Autodesk Fusion 360 part; units mm, degrees
(part 2 of 10)
sketch "Sketch15" plane through (0, 0, 9) normal (0, 0, 1) x (-1, 0, 0)
  line L0 (-13.7, 38.77) -> (-13.7, 37.77)
  line L1 (-13.7, 37.77) -> (-14.7, 37.77)
  line L2 (-14.7, 37.77) -> (-14.7, 38.77)
  line L3 (-14.7, 38.77) -> (-13.7, 38.77)
  line L4 (-13.7, 36.14) -> (-13.7, 35.14)
  line L5 (-13.7, 35.14) -> (-14.7, 35.14)
  line L6 (-14.7, 35.14) -> (-14.7, 36.14)
  line L7 (-14.7, 36.14) -> (-13.7, 36.14)
  line L8 (-13.7, 33.51) -> (-13.7, 32.51)
  line L9 (-13.7, 32.51) -> (-14.7, 32.51)
  line L10 (-14.7, 32.51) -> (-14.7, 33.51)
  line L11 (-14.7, 33.51) -> (-13.7, 33.51)
  line L12 (-13.7, 30.88) -> (-13.7, 29.88)
  line L13 (-13.7, 29.88) -> (-14.7, 29.88)
  line L14 (-14.7, 29.88) -> (-14.7, 30.88)
  line L15 (-14.7, 30.88) -> (-13.7, 30.88)
  line L16 (-13.7, 28.25) -> (-13.7, 27.25)
  line L17 (-13.7, 27.25) -> (-14.7, 27.25)
  line L18 (-14.7, 27.25) -> (-14.7, 28.25)
  line L19 (-14.7, 28.25) -> (-13.7, 28.25)
  line L20 (-13.7, 25.62) -> (-13.7, 24.62)
  line L21 (-13.7, 24.62) -> (-14.7, 24.62)
  line L22 (-14.7, 24.62) -> (-14.7, 25.62)
  line L23 (-14.7, 25.62) -> (-13.7, 25.62)
  line L24 (-13.7, 22.99) -> (-13.7, 21.99)
  line L25 (-13.7, 21.99) -> (-14.7, 21.99)
  line L26 (-14.7, 21.99) -> (-14.7, 22.99)
  line L27 (-14.7, 22.99) -> (-13.7, 22.99)
  line L28 (-13.7, 20.36) -> (-13.7, 19.36)
  line L29 (-13.7, 19.36) -> (-14.7, 19.36)
  line L30 (-14.7, 19.36) -> (-14.7, 20.36)
  line L31 (-14.7, 20.36) -> (-13.7, 20.36)
  line L32 (-13.7, 17.73) -> (-13.7, 16.73)
  line L33 (-13.7, 16.73) -> (-14.7, 16.73)
  line L34 (-14.7, 16.73) -> (-14.7, 17.73)
  line L35 (-14.7, 17.73) -> (-13.7, 17.73)
  line L36 (-13.7, 15.1) -> (-13.7, 14.1)
  line L37 (-13.7, 14.1) -> (-14.7, 14.1)
  line L38 (-14.7, 14.1) -> (-14.7, 15.1)
  line L39 (-14.7, 15.1) -> (-13.7, 15.1)
  line L40 (-13.7, 12.47) -> (-13.7, 11.47)
  line L41 (-13.7, 11.47) -> (-14.7, 11.47)
  line L42 (-14.7, 11.47) -> (-14.7, 12.47)
  line L43 (-14.7, 12.47) -> (-13.7, 12.47)
  line L44 (-13.7, 9.84) -> (-13.7, 8.84)
  line L45 (-13.7, 8.84) -> (-14.7, 8.84)
  line L46 (-14.7, 8.84) -> (-14.7, 9.84)
  line L47 (-14.7, 9.84) -> (-13.7, 9.84)
  line L48 (-13.7, 7.21) -> (-13.7, 6.21)
  line L49 (-13.7, 6.21) -> (-14.7, 6.21)
  line L50 (-14.7, 6.21) -> (-14.7, 7.21)
  line L51 (-14.7, 7.21) -> (-13.7, 7.21)
  line L52 (-13.7, 4.58) -> (-13.7, 3.58)
  line L53 (-13.7, 3.58) -> (-14.7, 3.58)
  line L54 (-14.7, 3.58) -> (-14.7, 4.58)
  line L55 (-14.7, 4.58) -> (-13.7, 4.58)
  line L56 (-13.7, 1.95) -> (-13.7, 0.95)
  line L57 (-13.7, 0.95) -> (-14.7, 0.95)
  line L58 (-14.7, 0.95) -> (-14.7, 1.95)
  line L59 (-14.7, 1.95) -> (-13.7, 1.95)
  line L60 (-13.7, -0.68) -> (-13.7, -1.68)
  line L61 (-13.7, -1.68) -> (-14.7, -1.68)
  line L62 (-14.7, -1.68) -> (-14.7, -0.68)
  line L63 (-14.7, -0.68) -> (-13.7, -0.68)
  line L64 (-13.7, -3.31) -> (-13.7, -4.31)
  line L65 (-13.7, -4.31) -> (-14.7, -4.31)
  line L66 (-14.7, -4.31) -> (-14.7, -3.31)
  line L67 (-14.7, -3.31) -> (-13.7, -3.31)
  line L68 (-13.7, -5.94) -> (-13.7, -6.94)
  line L69 (-13.7, -6.94) -> (-14.7, -6.94)
  line L70 (-14.7, -6.94) -> (-14.7, -5.94)
  line L71 (-14.7, -5.94) -> (-13.7, -5.94)
  line L72 (-13.7, -8.57) -> (-13.7, -9.57)
  line L73 (-13.7, -9.57) -> (-14.7, -9.57)
  line L74 (-14.7, -9.57) -> (-14.7, -8.57)
  line L75 (-14.7, -8.57) -> (-13.7, -8.57)
  line L76 (-13.7, -11.2) -> (-13.7, -12.2)
  line L77 (-13.7, -12.2) -> (-14.7, -12.2)
  line L78 (-14.7, -12.2) -> (-14.7, -11.2)
  line L79 (-14.7, -11.2) -> (-13.7, -11.2)
  line L80 (-13.7, -13.83) -> (-13.7, -14.83)
  line L81 (-13.7, -14.83) -> (-14.7, -14.83)
  line L82 (-14.7, -14.83) -> (-14.7, -13.83)
  line L83 (-14.7, -13.83) -> (-13.7, -13.83)
  line L84 (-13.7, -16.46) -> (-13.7, -17.46)
  line L85 (-13.7, -17.46) -> (-14.7, -17.46)
  line L86 (-14.7, -17.46) -> (-14.7, -16.46)
  line L87 (-14.7, -16.46) -> (-13.7, -16.46)
  line L88 (-13.7, -19.09) -> (-13.7, -20.09)
  line L89 (-13.7, -20.09) -> (-14.7, -20.09)
  line L90 (-14.7, -20.09) -> (-14.7, -19.09)
  line L91 (-14.7, -19.09) -> (-13.7, -19.09)
  line L92 (-13.7, -21.72) -> (-13.7, -22.72)
  line L93 (-13.7, -22.72) -> (-14.7, -22.72)
  line L94 (-14.7, -22.72) -> (-14.7, -21.72)
  line L95 (-14.7, -21.72) -> (-13.7, -21.72)
  line L96 (-13.7, -24.35) -> (-13.7, -25.35)
  line L97 (-13.7, -25.35) -> (-14.7, -25.35)
  line L98 (-14.7, -25.35) -> (-14.7, -24.35)
  line L99 (-14.7, -24.35) -> (-13.7, -24.35)
  line L100 (-13.7, -26.98) -> (-13.7, -27.98)
  line L101 (-13.7, -27.98) -> (-14.7, -27.98)
  line L102 (-14.7, -27.98) -> (-14.7, -26.98)
  line L103 (-14.7, -26.98) -> (-13.7, -26.98)
  line L104 (-13.7, -29.61) -> (-13.7, -30.61)
  line L105 (-13.7, -30.61) -> (-14.7, -30.61)
  line L106 (-14.7, -30.61) -> (-14.7, -29.61)
  line L107 (-14.7, -29.61) -> (-13.7, -29.61)
  line L108 (-13.7, -32.24) -> (-13.7, -33.24)
  line L109 (-13.7, -33.24) -> (-14.7, -33.24)
  line L110 (-14.7, -33.24) -> (-14.7, -32.24)
  line L111 (-14.7, -32.24) -> (-13.7, -32.24)
  line L112 (-13.7, -34.87) -> (-13.7, -35.87)
  line L113 (-13.7, -35.87) -> (-14.7, -35.87)
  line L114 (-14.7, -35.87) -> (-14.7, -34.87)
  line L115 (-14.7, -34.87) -> (-13.7, -34.87)
  line L116 (-13.7, -37.5) -> (-13.7, -38.5)
  line L117 (-13.7, -38.5) -> (-14.7, -38.5)
  line L118 (-14.7, -38.5) -> (-14.7, -37.5)
  line L119 (-14.7, -37.5) -> (-13.7, -37.5)
  line L120 (-10.9, 38.77) -> (-10.9, 37.77)
  line L121 (-10.9, 37.77) -> (-11.9, 37.77)
  line L122 (-11.9, 37.77) -> (-11.9, 38.77)
  line L123 (-11.9, 38.77) -> (-10.9, 38.77)
  line L124 (-10.9, 36.14) -> (-10.9, 35.14)
  line L125 (-10.9, 35.14) -> (-11.9, 35.14)
  line L126 (-11.9, 35.14) -> (-11.9, 36.14)
  line L127 (-11.9, 36.14) -> (-10.9, 36.14)
  line L128 (-10.9, 33.51) -> (-10.9, 32.51)
  line L129 (-10.9, 32.51) -> (-11.9, 32.51)
  line L130 (-11.9, 32.51) -> (-11.9, 33.51)
  line L131 (-11.9, 33.51) -> (-10.9, 33.51)
  line L132 (-10.9, 30.88) -> (-10.9, 29.88)
  line L133 (-10.9, 29.88) -> (-11.9, 29.88)
  line L134 (-11.9, 29.88) -> (-11.9, 30.88)
  line L135 (-11.9, 30.88) -> (-10.9, 30.88)
  line L136 (-10.9, 28.25) -> (-10.9, 27.25)
  line L137 (-10.9, 27.25) -> (-11.9, 27.25)
  line L138 (-11.9, 27.25) -> (-11.9, 28.25)
  line L139 (-11.9, 28.25) -> (-10.9, 28.25)
  line L140 (-10.9, 25.62) -> (-10.9, 24.62)
  line L141 (-10.9, 24.62) -> (-11.9, 24.62)
  line L142 (-11.9, 24.62) -> (-11.9, 25.62)
  line L143 (-11.9, 25.62) -> (-10.9, 25.62)
  line L144 (-10.9, 22.99) -> (-10.9, 21.99)
  line L145 (-10.9, 21.99) -> (-11.9, 21.99)
  line L146 (-11.9, 21.99) -> (-11.9, 22.99)
  line L147 (-11.9, 22.99) -> (-10.9, 22.99)
  line L148 (-10.9, 20.36) -> (-10.9, 19.36)
  line L149 (-10.9, 19.36) -> (-11.9, 19.36)
  line L150 (-11.9, 19.36) -> (-11.9, 20.36)
  line L151 (-11.9, 20.36) -> (-10.9, 20.36)
  line L152 (-10.9, 17.73) -> (-10.9, 16.73)
  line L153 (-10.9, 16.73) -> (-11.9, 16.73)
  line L154 (-11.9, 16.73) -> (-11.9, 17.73)
  line L155 (-11.9, 17.73) -> (-10.9, 17.73)
  line L156 (-10.9, 15.1) -> (-10.9, 14.1)
  line L157 (-10.9, 14.1) -> (-11.9, 14.1)
  line L158 (-11.9, 14.1) -> (-11.9, 15.1)
  line L159 (-11.9, 15.1) -> (-10.9, 15.1)
  line L160 (-10.9, 12.47) -> (-10.9, 11.47)
  line L161 (-10.9, 11.47) -> (-11.9, 11.47)
  line L162 (-11.9, 11.47) -> (-11.9, 12.47)
  line L163 (-11.9, 12.47) -> (-10.9, 12.47)
  line L164 (-10.9, 9.84) -> (-10.9, 8.84)
  line L165 (-10.9, 8.84) -> (-11.9, 8.84)
  line L166 (-11.9, 8.84) -> (-11.9, 9.84)
  line L167 (-11.9, 9.84) -> (-10.9, 9.84)
  line L168 (-10.9, 7.21) -> (-10.9, 6.21)
  line L169 (-10.9, 6.21) -> (-11.9, 6.21)
  line L170 (-11.9, 6.21) -> (-11.9, 7.21)
  line L171 (-11.9, 7.21) -> (-10.9, 7.21)
  line L172 (-10.9, 4.58) -> (-10.9, 3.58)
  line L173 (-10.9, 3.58) -> (-11.9, 3.58)
  line L174 (-11.9, 3.58) -> (-11.9, 4.58)
  line L175 (-11.9, 4.58) -> (-10.9, 4.58)
  line L176 (-10.9, 1.95) -> (-10.9, 0.95)
  line L177 (-10.9, 0.95) -> (-11.9, 0.95)
  line L178 (-11.9, 0.95) -> (-11.9, 1.95)
  line L179 (-11.9, 1.95) -> (-10.9, 1.95)
  line L180 (-10.9, -0.68) -> (-10.9, -1.68)
  line L181 (-10.9, -1.68) -> (-11.9, -1.68)
  line L182 (-11.9, -1.68) -> (-11.9, -0.68)
  line L183 (-11.9, -0.68) -> (-10.9, -0.68)
  line L184 (-10.9, -3.31) -> (-10.9, -4.31)
  line L185 (-10.9, -4.31) -> (-11.9, -4.31)
  line L186 (-11.9, -4.31) -> (-11.9, -3.31)
  line L187 (-11.9, -3.31) -> (-10.9, -3.31)
  line L188 (-10.9, -5.94) -> (-10.9, -6.94)
  line L189 (-10.9, -6.94) -> (-11.9, -6.94)
  line L190 (-11.9, -6.94) -> (-11.9, -5.94)
  line L191 (-11.9, -5.94) -> (-10.9, -5.94)
  line L192 (-10.9, -8.57) -> (-10.9, -9.57)
  line L193 (-10.9, -9.57) -> (-11.9, -9.57)
  line L194 (-11.9, -9.57) -> (-11.9, -8.57)
  line L195 (-11.9, -8.57) -> (-10.9, -8.57)
  line L196 (-10.9, -11.2) -> (-10.9, -12.2)
  line L197 (-10.9, -12.2) -> (-11.9, -12.2)
  line L198 (-11.9, -12.2) -> (-11.9, -11.2)
  line L199 (-11.9, -11.2) -> (-10.9, -11.2)
  line L200 (-10.9, -13.83) -> (-10.9, -14.83)
  line L201 (-10.9, -14.83) -> (-11.9, -14.83)
  line L202 (-11.9, -14.83) -> (-11.9, -13.83)
  line L203 (-11.9, -13.83) -> (-10.9, -13.83)
  line L204 (-10.9, -16.46) -> (-10.9, -17.46)
  line L205 (-10.9, -17.46) -> (-11.9, -17.46)
  line L206 (-11.9, -17.46) -> (-11.9, -16.46)
  line L207 (-11.9, -16.46) -> (-10.9, -16.46)
  line L208 (-10.9, -19.09) -> (-10.9, -20.09)
  line L209 (-10.9, -20.09) -> (-11.9, -20.09)
  line L210 (-11.9, -20.09) -> (-11.9, -19.09)
  line L211 (-11.9, -19.09) -> (-10.9, -19.09)
  line L212 (-10.9, -21.72) -> (-10.9, -22.72)
  line L213 (-10.9, -22.72) -> (-11.9, -22.72)
  line L214 (-11.9, -22.72) -> (-11.9, -21.72)
  line L215 (-11.9, -21.72) -> (-10.9, -21.72)
  line L216 (-10.9, -24.35) -> (-10.9, -25.35)
  line L217 (-10.9, -25.35) -> (-11.9, -25.35)
  line L218 (-11.9, -25.35) -> (-11.9, -24.35)
  line L219 (-11.9, -24.35) -> (-10.9, -24.35)
  line L220 (-10.9, -26.98) -> (-10.9, -27.98)
  line L221 (-10.9, -27.98) -> (-11.9, -27.98)
  line L222 (-11.9, -27.98) -> (-11.9, -26.98)
  line L223 (-11.9, -26.98) -> (-10.9, -26.98)
  line L224 (-10.9, -29.61) -> (-10.9, -30.61)
  line L225 (-10.9, -30.61) -> (-11.9, -30.61)
  line L226 (-11.9, -30.61) -> (-11.9, -29.61)
  line L227 (-11.9, -29.61) -> (-10.9, -29.61)
  line L228 (-10.9, -32.24) -> (-10.9, -33.24)
  line L229 (-10.9, -33.24) -> (-11.9, -33.24)
  line L230 (-11.9, -33.24) -> (-11.9, -32.24)
  line L231 (-11.9, -32.24) -> (-10.9, -32.24)
  line L232 (-10.9, -34.87) -> (-10.9, -35.87)
  line L233 (-10.9, -35.87) -> (-11.9, -35.87)
  line L234 (-11.9, -35.87) -> (-11.9, -34.87)
  line L235 (-11.9, -34.87) -> (-10.9, -34.87)
  line L236 (-10.9, -37.5) -> (-10.9, -38.5)
  line L237 (-10.9, -38.5) -> (-11.9, -38.5)
  line L238 (-11.9, -38.5) -> (-11.9, -37.5)
  line L239 (-11.9, -37.5) -> (-10.9, -37.5)
  line L240 (-8.1, 38.77) -> (-8.1, 37.77)
  line L241 (-8.1, 37.77) -> (-9.1, 37.77)
  line L242 (-9.1, 37.77) -> (-9.1, 38.77)
  line L243 (-9.1, 38.77) -> (-8.1, 38.77)
  line L244 (-8.1, 36.14) -> (-8.1, 35.14)
  line L245 (-8.1, 35.14) -> (-9.1, 35.14)
  line L246 (-9.1, 35.14) -> (-9.1, 36.14)
  line L247 (-9.1, 36.14) -> (-8.1, 36.14)
  line L248 (-8.1, 33.51) -> (-8.1, 32.51)
  line L249 (-8.1, 32.51) -> (-9.1, 32.51)
  line L250 (-9.1, 32.51) -> (-9.1, 33.51)
  line L251 (-9.1, 33.51) -> (-8.1, 33.51)
  line L252 (-8.1, 30.88) -> (-8.1, 29.88)
  line L253 (-8.1, 29.88) -> (-9.1, 29.88)
  line L254 (-9.1, 29.88) -> (-9.1, 30.88)
  line L255 (-9.1, 30.88) -> (-8.1, 30.88)
  line L256 (-8.1, 28.25) -> (-8.1, 27.25)
  line L257 (-8.1, 27.25) -> (-9.1, 27.25)
  line L258 (-9.1, 27.25) -> (-9.1, 28.25)
  line L259 (-9.1, 28.25) -> (-8.1, 28.25)
  line L260 (-8.1, 25.62) -> (-8.1, 24.62)
  line L261 (-8.1, 24.62) -> (-9.1, 24.62)
  line L262 (-9.1, 24.62) -> (-9.1, 25.62)
  line L263 (-9.1, 25.62) -> (-8.1, 25.62)
  line L264 (-8.1, 22.99) -> (-8.1, 21.99)
  line L265 (-8.1, 21.99) -> (-9.1, 21.99)
  line L266 (-9.1, 21.99) -> (-9.1, 22.99)
  line L267 (-9.1, 22.99) -> (-8.1, 22.99)
  line L268 (-8.1, 20.36) -> (-8.1, 19.36)
  line L269 (-8.1, 19.36) -> (-9.1, 19.36)
  line L270 (-9.1, 19.36) -> (-9.1, 20.36)
  line L271 (-9.1, 20.36) -> (-8.1, 20.36)
  line L272 (-8.1, 17.73) -> (-8.1, 16.73)
  line L273 (-8.1, 16.73) -> (-9.1, 16.73)
  line L274 (-9.1, 16.73) -> (-9.1, 17.73)
  line L275 (-9.1, 17.73) -> (-8.1, 17.73)
  line L276 (-8.1, 15.1) -> (-8.1, 14.1)
  line L277 (-8.1, 14.1) -> (-9.1, 14.1)
  line L278 (-9.1, 14.1) -> (-9.1, 15.1)
  line L279 (-9.1, 15.1) -> (-8.1, 15.1)
  line L280 (-8.1, 12.47) -> (-8.1, 11.47)
  line L281 (-8.1, 11.47) -> (-9.1, 11.47)
  line L282 (-9.1, 11.47) -> (-9.1, 12.47)
  line L283 (-9.1, 12.47) -> (-8.1, 12.47)
  line L284 (-8.1, 9.84) -> (-8.1, 8.84)
  line L285 (-8.1, 8.84) -> (-9.1, 8.84)
  line L286 (-9.1, 8.84) -> (-9.1, 9.84)
  line L287 (-9.1, 9.84) -> (-8.1, 9.84)
  line L288 (-8.1, 7.21) -> (-8.1, 6.21)
  line L289 (-8.1, 6.21) -> (-9.1, 6.21)
  line L290 (-9.1, 6.21) -> (-9.1, 7.21)
  line L291 (-9.1, 7.21) -> (-8.1, 7.21)
  line L292 (-8.1, 4.58) -> (-8.1, 3.58)
  line L293 (-8.1, 3.58) -> (-9.1, 3.58)
  line L294 (-9.1, 3.58) -> (-9.1, 4.58)
  line L295 (-9.1, 4.58) -> (-8.1, 4.58)
  line L296 (-8.1, 1.95) -> (-8.1, 0.95)
  line L297 (-8.1, 0.95) -> (-9.1, 0.95)
  line L298 (-9.1, 0.95) -> (-9.1, 1.95)
  line L299 (-9.1, 1.95) -> (-8.1, 1.95)
  line L300 (-8.1, -0.68) -> (-8.1, -1.68)
  line L301 (-8.1, -1.68) -> (-9.1, -1.68)
  line L302 (-9.1, -1.68) -> (-9.1, -0.68)
  line L303 (-9.1, -0.68) -> (-8.1, -0.68)
  line L304 (-8.1, -3.31) -> (-8.1, -4.31)
  line L305 (-8.1, -4.31) -> (-9.1, -4.31)
  line L306 (-9.1, -4.31) -> (-9.1, -3.31)
  line L307 (-9.1, -3.31) -> (-8.1, -3.31)
  line L308 (-8.1, -5.94) -> (-8.1, -6.94)
  line L309 (-8.1, -6.94) -> (-9.1, -6.94)
  line L310 (-9.1, -6.94) -> (-9.1, -5.94)
  line L311 (-9.1, -5.94) -> (-8.1, -5.94)
  line L312 (-8.1, -8.57) -> (-8.1, -9.57)
  line L313 (-8.1, -9.57) -> (-9.1, -9.57)
  line L314 (-9.1, -9.57) -> (-9.1, -8.57)
  line L315 (-9.1, -8.57) -> (-8.1, -8.57)
  line L316 (-8.1, -11.2) -> (-8.1, -12.2)
  line L317 (-8.1, -12.2) -> (-9.1, -12.2)
  line L318 (-9.1, -12.2) -> (-9.1, -11.2)
  line L319 (-9.1, -11.2) -> (-8.1, -11.2)
  line L320 (-8.1, -13.83) -> (-8.1, -14.83)
  line L321 (-8.1, -14.83) -> (-9.1, -14.83)
  line L322 (-9.1, -14.83) -> (-9.1, -13.83)
  line L323 (-9.1, -13.83) -> (-8.1, -13.83)
  line L324 (-8.1, -16.46) -> (-8.1, -17.46)
  line L325 (-8.1, -17.46) -> (-9.1, -17.46)
  line L326 (-9.1, -17.46) -> (-9.1, -16.46)
  line L327 (-9.1, -16.46) -> (-8.1, -16.46)
  line L328 (-8.1, -19.09) -> (-8.1, -20.09)
  line L329 (-8.1, -20.09) -> (-9.1, -20.09)
  line L330 (-9.1, -20.09) -> (-9.1, -19.09)
  line L331 (-9.1, -19.09) -> (-8.1, -19.09)
  line L332 (-8.1, -21.72) -> (-8.1, -22.72)
  line L333 (-8.1, -22.72) -> (-9.1, -22.72)
  line L334 (-9.1, -22.72) -> (-9.1, -21.72)
  line L335 (-9.1, -21.72) -> (-8.1, -21.72)
  line L336 (-8.1, -24.35) -> (-8.1, -25.35)
  line L337 (-8.1, -25.35) -> (-9.1, -25.35)
  line L338 (-9.1, -25.35) -> (-9.1, -24.35)
  line L339 (-9.1, -24.35) -> (-8.1, -24.35)
  line L340 (-8.1, -26.98) -> (-8.1, -27.98)
  line L341 (-8.1, -27.98) -> (-9.1, -27.98)
  line L342 (-9.1, -27.98) -> (-9.1, -26.98)
  line L343 (-9.1, -26.98) -> (-8.1, -26.98)
  line L344 (-8.1, -29.61) -> (-8.1, -30.61)
  line L345 (-8.1, -30.61) -> (-9.1, -30.61)
  line L346 (-9.1, -30.61) -> (-9.1, -29.61)
  line L347 (-9.1, -29.61) -> (-8.1, -29.61)
  line L348 (-8.1, -32.24) -> (-8.1, -33.24)
  line L349 (-8.1, -33.24) -> (-9.1, -33.24)
  line L350 (-9.1, -33.24) -> (-9.1, -32.24)
  line L351 (-9.1, -32.24) -> (-8.1, -32.24)
  line L352 (-8.1, -34.87) -> (-8.1, -35.87)
  line L353 (-8.1, -35.87) -> (-9.1, -35.87)
  line L354 (-9.1, -35.87) -> (-9.1, -34.87)
  line L355 (-9.1, -34.87) -> (-8.1, -34.87)
  line L356 (-8.1, -37.5) -> (-8.1, -38.5)
  line L357 (-8.1, -38.5) -> (-9.1, -38.5)
  line L358 (-9.1, -38.5) -> (-9.1, -37.5)
  line L359 (-9.1, -37.5) -> (-8.1, -37.5)
  line L360 (-5.3, 38.77) -> (-5.3, 37.77)
  line L361 (-5.3, 37.77) -> (-6.3, 37.77)
  line L362 (-6.3, 37.77) -> (-6.3, 38.77)
  line L363 (-6.3, 38.77) -> (-5.3, 38.77)
  line L364 (-5.3, 36.14) -> (-5.3, 35.14)
  line L365 (-5.3, 35.14) -> (-6.3, 35.14)
  line L366 (-6.3, 35.14) -> (-6.3, 36.14)
  line L367 (-6.3, 36.14) -> (-5.3, 36.14)
  line L368 (-5.3, 33.51) -> (-5.3, 32.51)
  line L369 (-5.3, 32.51) -> (-6.3, 32.51)
  line L370 (-6.3, 32.51) -> (-6.3, 33.51)
  line L371 (-6.3, 33.51) -> (-5.3, 33.51)
  line L372 (-5.3, 30.88) -> (-5.3, 29.88)
  line L373 (-5.3, 29.88) -> (-6.3, 29.88)
  line L374 (-6.3, 29.88) -> (-6.3, 30.88)
  line L375 (-6.3, 30.88) -> (-5.3, 30.88)
  line L376 (-5.3, 28.25) -> (-5.3, 27.25)
  line L377 (-5.3, 27.25) -> (-6.3, 27.25)
  line L378 (-6.3, 27.25) -> (-6.3, 28.25)
  line L379 (-6.3, 28.25) -> (-5.3, 28.25)
  line L380 (-5.3, 25.62) -> (-5.3, 24.62)
  line L381 (-5.3, 24.62) -> (-6.3, 24.62)
  line L382 (-6.3, 24.62) -> (-6.3, 25.62)
  line L383 (-6.3, 25.62) -> (-5.3, 25.62)
  line L384 (-5.3, 22.99) -> (-5.3, 21.99)
  line L385 (-5.3, 21.99) -> (-6.3, 21.99)
  line L386 (-6.3, 21.99) -> (-6.3, 22.99)
  line L387 (-6.3, 22.99) -> (-5.3, 22.99)
  line L388 (-5.3, 20.36) -> (-5.3, 19.36)
  line L389 (-5.3, 19.36) -> (-6.3, 19.36)
  line L390 (-6.3, 19.36) -> (-6.3, 20.36)
  line L391 (-6.3, 20.36) -> (-5.3, 20.36)
  line L392 (-5.3, 17.73) -> (-5.3, 16.73)
  line L393 (-5.3, 16.73) -> (-6.3, 16.73)
  line L394 (-6.3, 16.73) -> (-6.3, 17.73)
  line L395 (-6.3, 17.73) -> (-5.3, 17.73)
  line L396 (-5.3, 15.1) -> (-5.3, 14.1)
  line L397 (-5.3, 14.1) -> (-6.3, 14.1)
  line L398 (-6.3, 14.1) -> (-6.3, 15.1)
  line L399 (-6.3, 15.1) -> (-5.3, 15.1)
  line L400 (-5.3, 12.47) -> (-5.3, 11.47)
  line L401 (-5.3, 11.47) -> (-6.3, 11.47)
  line L402 (-6.3, 11.47) -> (-6.3, 12.47)
  line L403 (-6.3, 12.47) -> (-5.3, 12.47)
  line L404 (-5.3, 9.84) -> (-5.3, 8.84)
  line L405 (-5.3, 8.84) -> (-6.3, 8.84)
  line L406 (-6.3, 8.84) -> (-6.3, 9.84)
  line L407 (-6.3, 9.84) -> (-5.3, 9.84)
  line L408 (-5.3, 7.21) -> (-5.3, 6.21)
  line L409 (-5.3, 6.21) -> (-6.3, 6.21)
  line L410 (-6.3, 6.21) -> (-6.3, 7.21)
  line L411 (-6.3, 7.21) -> (-5.3, 7.21)
  line L412 (-5.3, 4.58) -> (-5.3, 3.58)
  line L413 (-5.3, 3.58) -> (-6.3, 3.58)
  line L414 (-6.3, 3.58) -> (-6.3, 4.58)
  line L415 (-6.3, 4.58) -> (-5.3, 4.58)
  line L416 (-5.3, 1.95) -> (-5.3, 0.95)
  line L417 (-5.3, 0.95) -> (-6.3, 0.95)
  line L418 (-6.3, 0.95) -> (-6.3, 1.95)
  line L419 (-6.3, 1.95) -> (-5.3, 1.95)
  line L420 (-5.3, -0.68) -> (-5.3, -1.68)
  line L421 (-5.3, -1.68) -> (-6.3, -1.68)
  line L422 (-6.3, -1.68) -> (-6.3, -0.68)
  line L423 (-6.3, -0.68) -> (-5.3, -0.68)
  line L424 (-5.3, -3.31) -> (-5.3, -4.31)
  line L425 (-5.3, -4.31) -> (-6.3, -4.31)
  line L426 (-6.3, -4.31) -> (-6.3, -3.31)
  line L427 (-6.3, -3.31) -> (-5.3, -3.31)
  line L428 (-5.3, -5.94) -> (-5.3, -6.94)
  line L429 (-5.3, -6.94) -> (-6.3, -6.94)
  line L430 (-6.3, -6.94) -> (-6.3, -5.94)
  line L431 (-6.3, -5.94) -> (-5.3, -5.94)
  line L432 (-5.3, -8.57) -> (-5.3, -9.57)
  line L433 (-5.3, -9.57) -> (-6.3, -9.57)
  line L434 (-6.3, -9.57) -> (-6.3, -8.57)
  line L435 (-6.3, -8.57) -> (-5.3, -8.57)
  line L436 (-5.3, -11.2) -> (-5.3, -12.2)
  line L437 (-5.3, -12.2) -> (-6.3, -12.2)
  line L438 (-6.3, -12.2) -> (-6.3, -11.2)
  line L439 (-6.3, -11.2) -> (-5.3, -11.2)
  line L440 (-5.3, -13.83) -> (-5.3, -14.83)
  line L441 (-5.3, -14.83) -> (-6.3, -14.83)
  line L442 (-6.3, -14.83) -> (-6.3, -13.83)
  line L443 (-6.3, -13.83) -> (-5.3, -13.83)
  line L444 (-5.3, -16.46) -> (-5.3, -17.46)
  line L445 (-5.3, -17.46) -> (-6.3, -17.46)
  line L446 (-6.3, -17.46) -> (-6.3, -16.46)
  line L447 (-6.3, -16.46) -> (-5.3, -16.46)
  line L448 (-5.3, -19.09) -> (-5.3, -20.09)
  line L449 (-5.3, -20.09) -> (-6.3, -20.09)
  line L450 (-6.3, -20.09) -> (-6.3, -19.09)
  line L451 (-6.3, -19.09) -> (-5.3, -19.09)
  line L452 (-5.3, -21.72) -> (-5.3, -22.72)
  line L453 (-5.3, -22.72) -> (-6.3, -22.72)
  line L454 (-6.3, -22.72) -> (-6.3, -21.72)
  line L455 (-6.3, -21.72) -> (-5.3, -21.72)
  line L456 (-5.3, -24.35) -> (-5.3, -25.35)
  line L457 (-5.3, -25.35) -> (-6.3, -25.35)
  line L458 (-6.3, -25.35) -> (-6.3, -24.35)
  line L459 (-6.3, -24.35) -> (-5.3, -24.35)
  line L460 (-5.3, -26.98) -> (-5.3, -27.98)
  line L461 (-5.3, -27.98) -> (-6.3, -27.98)
  line L462 (-6.3, -27.98) -> (-6.3, -26.98)
  line L463 (-6.3, -26.98) -> (-5.3, -26.98)
  line L464 (-5.3, -29.61) -> (-5.3, -30.61)
  line L465 (-5.3, -30.61) -> (-6.3, -30.61)
  line L466 (-6.3, -30.61) -> (-6.3, -29.61)
  line L467 (-6.3, -29.61) -> (-5.3, -29.61)
  line L468 (-5.3, -32.24) -> (-5.3, -33.24)
  line L469 (-5.3, -33.24) -> (-6.3, -33.24)
  line L470 (-6.3, -33.24) -> (-6.3, -32.24)
  line L471 (-6.3, -32.24) -> (-5.3, -32.24)
  line L472 (-5.3, -34.87) -> (-5.3, -35.87)
  line L473 (-5.3, -35.87) -> (-6.3, -35.87)
  line L474 (-6.3, -35.87) -> (-6.3, -34.87)
  line L475 (-6.3, -34.87) -> (-5.3, -34.87)
  line L476 (-5.3, -37.5) -> (-5.3, -38.5)
  line L477 (-5.3, -38.5) -> (-6.3, -38.5)
  line L478 (-6.3, -38.5) -> (-6.3, -37.5)
  line L479 (-6.3, -37.5) -> (-5.3, -37.5)
  line L480 (-2.5, 38.77) -> (-2.5, 37.77)
  line L481 (-2.5, 37.77) -> (-3.5, 37.77)
  line L482 (-3.5, 37.77) -> (-3.5, 38.77)
  line L483 (-3.5, 38.77) -> (-2.5, 38.77)
  line L484 (-2.5, 36.14) -> (-2.5, 35.14)
  line L485 (-2.5, 35.14) -> (-3.5, 35.14)
  line L486 (-3.5, 35.14) -> (-3.5, 36.14)
  line L487 (-3.5, 36.14) -> (-2.5, 36.14)
  line L488 (-2.5, 33.51) -> (-2.5, 32.51)
  line L489 (-2.5, 32.51) -> (-3.5, 32.51)
  line L490 (-3.5, 32.51) -> (-3.5, 33.51)
  line L491 (-3.5, 33.51) -> (-2.5, 33.51)
  line L492 (-2.5, 30.88) -> (-2.5, 29.88)
  line L493 (-2.5, 29.88) -> (-3.5, 29.88)
  line L494 (-3.5, 29.88) -> (-3.5, 30.88)
  line L495 (-3.5, 30.88) -> (-2.5, 30.88)
  line L496 (-2.5, 28.25) -> (-2.5, 27.25)
  line L497 (-2.5, 27.25) -> (-3.5, 27.25)
  line L498 (-3.5, 27.25) -> (-3.5, 28.25)
  line L499 (-3.5, 28.25) -> (-2.5, 28.25)
  line L500 (-2.5, 25.62) -> (-2.5, 24.62)
  line L501 (-2.5, 24.62) -> (-3.5, 24.62)
  line L502 (-3.5, 24.62) -> (-3.5, 25.62)
  line L503 (-3.5, 25.62) -> (-2.5, 25.62)
  line L504 (-2.5, 22.99) -> (-2.5, 21.99)
  line L505 (-2.5, 21.99) -> (-3.5, 21.99)
  line L506 (-3.5, 21.99) -> (-3.5, 22.99)
  line L507 (-3.5, 22.99) -> (-2.5, 22.99)
  line L508 (-2.5, 20.36) -> (-2.5, 19.36)
  line L509 (-2.5, 19.36) -> (-3.5, 19.36)
  line L510 (-3.5, 19.36) -> (-3.5, 20.36)
  line L511 (-3.5, 20.36) -> (-2.5, 20.36)
  line L512 (-2.5, 17.73) -> (-2.5, 16.73)
  line L513 (-2.5, 16.73) -> (-3.5, 16.73)
  line L514 (-3.5, 16.73) -> (-3.5, 17.73)
  line L515 (-3.5, 17.73) -> (-2.5, 17.73)
  line L516 (-2.5, 15.1) -> (-2.5, 14.1)
  line L517 (-2.5, 14.1) -> (-3.5, 14.1)
  line L518 (-3.5, 14.1) -> (-3.5, 15.1)
  line L519 (-3.5, 15.1) -> (-2.5, 15.1)
  line L520 (-2.5, 12.47) -> (-2.5, 11.47)
  line L521 (-2.5, 11.47) -> (-3.5, 11.47)
  line L522 (-3.5, 11.47) -> (-3.5, 12.47)
  line L523 (-3.5, 12.47) -> (-2.5, 12.47)
  line L524 (-2.5, 9.84) -> (-2.5, 8.84)
  line L525 (-2.5, 8.84) -> (-3.5, 8.84)
  line L526 (-3.5, 8.84) -> (-3.5, 9.84)
  line L527 (-3.5, 9.84) -> (-2.5, 9.84)
  line L528 (-2.5, 7.21) -> (-2.5, 6.21)
  line L529 (-2.5, 6.21) -> (-3.5, 6.21)
  line L530 (-3.5, 6.21) -> (-3.5, 7.21)
  line L531 (-3.5, 7.21) -> (-2.5, 7.21)
  line L532 (-2.5, 4.58) -> (-2.5, 3.58)
  line L533 (-2.5, 3.58) -> (-3.5, 3.58)
  line L534 (-3.5, 3.58) -> (-3.5, 4.58)
  line L535 (-3.5, 4.58) -> (-2.5, 4.58)
  line L536 (-2.5, 1.95) -> (-2.5, 0.95)
  line L537 (-2.5, 0.95) -> (-3.5, 0.95)
  line L538 (-3.5, 0.95) -> (-3.5, 1.95)
  line L539 (-3.5, 1.95) -> (-2.5, 1.95)
  line L540 (-2.5, -0.68) -> (-2.5, -1.68)
  line L541 (-2.5, -1.68) -> (-3.5, -1.68)
  line L542 (-3.5, -1.68) -> (-3.5, -0.68)
  line L543 (-3.5, -0.68) -> (-2.5, -0.68)
  line L544 (-2.5, -3.31) -> (-2.5, -4.31)
  line L545 (-2.5, -4.31) -> (-3.5, -4.31)
  line L546 (-3.5, -4.31) -> (-3.5, -3.31)
  line L547 (-3.5, -3.31) -> (-2.5, -3.31)
  line L548 (-2.5, -5.94) -> (-2.5, -6.94)
  line L549 (-2.5, -6.94) -> (-3.5, -6.94)
  line L550 (-3.5, -6.94) -> (-3.5, -5.94)
  line L551 (-3.5, -5.94) -> (-2.5, -5.94)
  line L552 (-2.5, -8.57) -> (-2.5, -9.57)
  line L553 (-2.5, -9.57) -> (-3.5, -9.57)
  line L554 (-3.5, -9.57) -> (-3.5, -8.57)
  line L555 (-3.5, -8.57) -> (-2.5, -8.57)
  line L556 (-2.5, -11.2) -> (-2.5, -12.2)
  line L557 (-2.5, -12.2) -> (-3.5, -12.2)
  line L558 (-3.5, -12.2) -> (-3.5, -11.2)
  line L559 (-3.5, -11.2) -> (-2.5, -11.2)
  line L560 (-2.5, -13.83) -> (-2.5, -14.83)
  line L561 (-2.5, -14.83) -> (-3.5, -14.83)
  line L562 (-3.5, -14.83) -> (-3.5, -13.83)
  line L563 (-3.5, -13.83) -> (-2.5, -13.83)
  line L564 (-2.5, -16.46) -> (-2.5, -17.46)
  line L565 (-2.5, -17.46) -> (-3.5, -17.46)
  line L566 (-3.5, -17.46) -> (-3.5, -16.46)
  line L567 (-3.5, -16.46) -> (-2.5, -16.46)
  line L568 (-2.5, -19.09) -> (-2.5, -20.09)
  line L569 (-2.5, -20.09) -> (-3.5, -20.09)
  line L570 (-3.5, -20.09) -> (-3.5, -19.09)
  line L571 (-3.5, -19.09) -> (-2.5, -19.09)
  line L572 (-2.5, -21.72) -> (-2.5, -22.72)
  line L573 (-2.5, -22.72) -> (-3.5, -22.72)
  line L574 (-3.5, -22.72) -> (-3.5, -21.72)
  line L575 (-3.5, -21.72) -> (-2.5, -21.72)
  line L576 (-2.5, -24.35) -> (-2.5, -25.35)
  line L577 (-2.5, -25.35) -> (-3.5, -25.35)
  line L578 (-3.5, -25.35) -> (-3.5, -24.35)
  line L579 (-3.5, -24.35) -> (-2.5, -24.35)
  line L580 (-2.5, -26.98) -> (-2.5, -27.98)
  line L581 (-2.5, -27.98) -> (-3.5, -27.98)
  line L582 (-3.5, -27.98) -> (-3.5, -26.98)
  line L583 (-3.5, -26.98) -> (-2.5, -26.98)
  line L584 (-2.5, -29.61) -> (-2.5, -30.61)
  line L585 (-2.5, -30.61) -> (-3.5, -30.61)
  line L586 (-3.5, -30.61) -> (-3.5, -29.61)
  line L587 (-3.5, -29.61) -> (-2.5, -29.61)
  line L588 (-2.5, -32.24) -> (-2.5, -33.24)
  line L589 (-2.5, -33.24) -> (-3.5, -33.24)
  line L590 (-3.5, -33.24) -> (-3.5, -32.24)
  line L591 (-3.5, -32.24) -> (-2.5, -32.24)
  line L592 (-2.5, -34.87) -> (-2.5, -35.87)
  line L593 (-2.5, -35.87) -> (-3.5, -35.87)
  line L594 (-3.5, -35.87) -> (-3.5, -34.87)
  line L595 (-3.5, -34.87) -> (-2.5, -34.87)
  line L596 (-2.5, -37.5) -> (-2.5, -38.5)
  line L597 (-2.5, -38.5) -> (-3.5, -38.5)
  line L598 (-3.5, -38.5) -> (-3.5, -37.5)
  line L599 (-3.5, -37.5) -> (-2.5, -37.5)
  line L600 (-1, -40.5) -> (-1, 40.5)
  line L601 (-1, 40.5) -> (-26.5, 40.5)
  line L602 (-26.5, 40.5) -> (-26.5, -40.5)
  line L603 (-26.5, -40.5) -> (-1, -40.5)
  line L604 (23, -35.5) -> (24, -35.5)
  line L605 (24, -35.5) -> (24, -36.5)
  line L606 (24, -36.5) -> (23, -36.5)
  line L607 (23, -36.5) -> (23, -35.5)
  line L608 (23, -35.5) -> (24, -36.5) construction
  line L609 (24, -35.5) -> (23, -36.5) construction
  line L610 (26.5, -40.5) -> (26.5, 40.5)
  line L611 (1, -40.5) -> (26.5, -40.5)
  point P0 (23.5, -36)
  dimension "d77" = 1
  dimension "d78" = 1
  dimension "d79" = 2.5
  dimension "d80" = 4
  constraint horizontal L604
  constraint perpendicular L604 L605
  constraint parallel L604 L606
  constraint parallel L605 L607
  constraint coincident L608 P0
  constraint coincident L609 P0
  measures "d77" distance of L605.end L606.end
  measures "d78" distance of L604.start L606.end
  measures "d79" distance of L605 L610
  measures "d80" distance of L606 L611
extrude "Extrude21" cut sketch "Sketch15" against normal blind 1 contours L604 L605 L606 L607 bodies 1
pattern_linear "R-Pattern3" count 2 spacing 3 along (1, 0, 0) count 5 spacing 2.63 along (0, -1, 0) of "Extrude21"
sketch "Sketch16" plane through (0, 0, 9) normal (0, 0, 1) x (-1, 0, 0)
  line L0 (-13.7, 38.77) -> (-13.7, 37.77)
  line L1 (-13.7, 37.77) -> (-14.7, 37.77)
  line L2 (-14.7, 37.77) -> (-14.7, 38.77)
  line L3 (-14.7, 38.77) -> (-13.7, 38.77)
  line L4 (-13.7, 36.14) -> (-13.7, 35.14)
  line L5 (-13.7, 35.14) -> (-14.7, 35.14)
  line L6 (-14.7, 35.14) -> (-14.7, 36.14)
  line L7 (-14.7, 36.14) -> (-13.7, 36.14)
  line L8 (-13.7, 33.51) -> (-13.7, 32.51)
  line L9 (-13.7, 32.51) -> (-14.7, 32.51)
  line L10 (-14.7, 32.51) -> (-14.7, 33.51)
  line L11 (-14.7, 33.51) -> (-13.7, 33.51)
  line L12 (-13.7, 30.88) -> (-13.7, 29.88)
  line L13 (-13.7, 29.88) -> (-14.7, 29.88)
  line L14 (-14.7, 29.88) -> (-14.7, 30.88)
  line L15 (-14.7, 30.88) -> (-13.7, 30.88)
  line L16 (-13.7, 28.25) -> (-13.7, 27.25)
  line L17 (-13.7, 27.25) -> (-14.7, 27.25)
  line L18 (-14.7, 27.25) -> (-14.7, 28.25)
  line L19 (-14.7, 28.25) -> (-13.7, 28.25)
  line L20 (-13.7, 25.62) -> (-13.7, 24.62)
  line L21 (-13.7, 24.62) -> (-14.7, 24.62)
  line L22 (-14.7, 24.62) -> (-14.7, 25.62)
  line L23 (-14.7, 25.62) -> (-13.7, 25.62)
  line L24 (-13.7, 22.99) -> (-13.7, 21.99)
  line L25 (-13.7, 21.99) -> (-14.7, 21.99)
  line L26 (-14.7, 21.99) -> (-14.7, 22.99)
  line L27 (-14.7, 22.99) -> (-13.7, 22.99)
  line L28 (-13.7, 20.36) -> (-13.7, 19.36)
  line L29 (-13.7, 19.36) -> (-14.7, 19.36)
  line L30 (-14.7, 19.36) -> (-14.7, 20.36)
  line L31 (-14.7, 20.36) -> (-13.7, 20.36)
  line L32 (-13.7, 17.73) -> (-13.7, 16.73)
  line L33 (-13.7, 16.73) -> (-14.7, 16.73)
  line L34 (-14.7, 16.73) -> (-14.7, 17.73)
  line L35 (-14.7, 17.73) -> (-13.7, 17.73)
  line L36 (-13.7, 15.1) -> (-13.7, 14.1)
  line L37 (-13.7, 14.1) -> (-14.7, 14.1)
  line L38 (-14.7, 14.1) -> (-14.7, 15.1)
  line L39 (-14.7, 15.1) -> (-13.7, 15.1)
  line L40 (-13.7, 12.47) -> (-13.7, 11.47)
  line L41 (-13.7, 11.47) -> (-14.7, 11.47)
  line L42 (-14.7, 11.47) -> (-14.7, 12.47)
  line L43 (-14.7, 12.47) -> (-13.7, 12.47)
  line L44 (-13.7, 9.84) -> (-13.7, 8.84)
  line L45 (-13.7, 8.84) -> (-14.7, 8.84)
  line L46 (-14.7, 8.84) -> (-14.7, 9.84)
  line L47 (-14.7, 9.84) -> (-13.7, 9.84)
  line L48 (-13.7, 7.21) -> (-13.7, 6.21)
  line L49 (-13.7, 6.21) -> (-14.7, 6.21)
  line L50 (-14.7, 6.21) -> (-14.7, 7.21)
  line L51 (-14.7, 7.21) -> (-13.7, 7.21)
  line L52 (-13.7, 4.58) -> (-13.7, 3.58)
  line L53 (-13.7, 3.58) -> (-14.7, 3.58)
  line L54 (-14.7, 3.58) -> (-14.7, 4.58)
  line L55 (-14.7, 4.58) -> (-13.7, 4.58)
  line L56 (-13.7, 1.95) -> (-13.7, 0.95)
  line L57 (-13.7, 0.95) -> (-14.7, 0.95)
  line L58 (-14.7, 0.95) -> (-14.7, 1.95)
  line L59 (-14.7, 1.95) -> (-13.7, 1.95)
  line L60 (-13.7, -0.68) -> (-13.7, -1.68)
  line L61 (-13.7, -1.68) -> (-14.7, -1.68)
  line L62 (-14.7, -1.68) -> (-14.7, -0.68)
  line L63 (-14.7, -0.68) -> (-13.7, -0.68)
  line L64 (-13.7, -3.31) -> (-13.7, -4.31)
  line L65 (-13.7, -4.31) -> (-14.7, -4.31)
  line L66 (-14.7, -4.31) -> (-14.7, -3.31)
  line L67 (-14.7, -3.31) -> (-13.7, -3.31)
  line L68 (-13.7, -5.94) -> (-13.7, -6.94)
  line L69 (-13.7, -6.94) -> (-14.7, -6.94)
  line L70 (-14.7, -6.94) -> (-14.7, -5.94)
  line L71 (-14.7, -5.94) -> (-13.7, -5.94)
  line L72 (-13.7, -8.57) -> (-13.7, -9.57)
  line L73 (-13.7, -9.57) -> (-14.7, -9.57)
  line L74 (-14.7, -9.57) -> (-14.7, -8.57)
  line L75 (-14.7, -8.57) -> (-13.7, -8.57)
  line L76 (-13.7, -11.2) -> (-13.7, -12.2)
  line L77 (-13.7, -12.2) -> (-14.7, -12.2)
  line L78 (-14.7, -12.2) -> (-14.7, -11.2)
  line L79 (-14.7, -11.2) -> (-13.7, -11.2)
  line L80 (-13.7, -13.83) -> (-13.7, -14.83)
  line L81 (-13.7, -14.83) -> (-14.7, -14.83)
  line L82 (-14.7, -14.83) -> (-14.7, -13.83)
  line L83 (-14.7, -13.83) -> (-13.7, -13.83)
  line L84 (-13.7, -16.46) -> (-13.7, -17.46)
  line L85 (-13.7, -17.46) -> (-14.7, -17.46)
  line L86 (-14.7, -17.46) -> (-14.7, -16.46)
  line L87 (-14.7, -16.46) -> (-13.7, -16.46)
  line L88 (-13.7, -19.09) -> (-13.7, -20.09)
  line L89 (-13.7, -20.09) -> (-14.7, -20.09)
  line L90 (-14.7, -20.09) -> (-14.7, -19.09)
  line L91 (-14.7, -19.09) -> (-13.7, -19.09)
  line L92 (-13.7, -21.72) -> (-13.7, -22.72)
  line L93 (-13.7, -22.72) -> (-14.7, -22.72)
  line L94 (-14.7, -22.72) -> (-14.7, -21.72)
  line L95 (-14.7, -21.72) -> (-13.7, -21.72)
  line L96 (-13.7, -24.35) -> (-13.7, -25.35)
  line L97 (-13.7, -25.35) -> (-14.7, -25.35)
  line L98 (-14.7, -25.35) -> (-14.7, -24.35)
  line L99 (-14.7, -24.35) -> (-13.7, -24.35)
  line L100 (-13.7, -26.98) -> (-13.7, -27.98)
  line L101 (-13.7, -27.98) -> (-14.7, -27.98)
  line L102 (-14.7, -27.98) -> (-14.7, -26.98)
  line L103 (-14.7, -26.98) -> (-13.7, -26.98)
  line L104 (-13.7, -29.61) -> (-13.7, -30.61)
  line L105 (-13.7, -30.61) -> (-14.7, -30.61)
  line L106 (-14.7, -30.61) -> (-14.7, -29.61)
  line L107 (-14.7, -29.61) -> (-13.7, -29.61)
  line L108 (-13.7, -32.24) -> (-13.7, -33.24)
  line L109 (-13.7, -33.24) -> (-14.7, -33.24)
  line L110 (-14.7, -33.24) -> (-14.7, -32.24)
  line L111 (-14.7, -32.24) -> (-13.7, -32.24)
  line L112 (-13.7, -34.87) -> (-13.7, -35.87)
  line L113 (-13.7, -35.87) -> (-14.7, -35.87)
  line L114 (-14.7, -35.87) -> (-14.7, -34.87)
  line L115 (-14.7, -34.87) -> (-13.7, -34.87)
  line L116 (-13.7, -37.5) -> (-13.7, -38.5)
  line L117 (-13.7, -38.5) -> (-14.7, -38.5)
  line L118 (-14.7, -38.5) -> (-14.7, -37.5)
  line L119 (-14.7, -37.5) -> (-13.7, -37.5)
  line L120 (-10.9, 38.77) -> (-10.9, 37.77)
  line L121 (-10.9, 37.77) -> (-11.9, 37.77)
  line L122 (-11.9, 37.77) -> (-11.9, 38.77)
  line L123 (-11.9, 38.77) -> (-10.9, 38.77)
  line L124 (-10.9, 36.14) -> (-10.9, 35.14)
  line L125 (-10.9, 35.14) -> (-11.9, 35.14)
  line L126 (-11.9, 35.14) -> (-11.9, 36.14)
  line L127 (-11.9, 36.14) -> (-10.9, 36.14)
  line L128 (-10.9, 33.51) -> (-10.9, 32.51)
  line L129 (-10.9, 32.51) -> (-11.9, 32.51)
  line L130 (-11.9, 32.51) -> (-11.9, 33.51)
  line L131 (-11.9, 33.51) -> (-10.9, 33.51)
  line L132 (-10.9, 30.88) -> (-10.9, 29.88)
  line L133 (-10.9, 29.88) -> (-11.9, 29.88)
  line L134 (-11.9, 29.88) -> (-11.9, 30.88)
  line L135 (-11.9, 30.88) -> (-10.9, 30.88)
  line L136 (-10.9, 28.25) -> (-10.9, 27.25)
  line L137 (-10.9, 27.25) -> (-11.9, 27.25)
  line L138 (-11.9, 27.25) -> (-11.9, 28.25)
  line L139 (-11.9, 28.25) -> (-10.9, 28.25)
  line L140 (-10.9, 25.62) -> (-10.9, 24.62)
  line L141 (-10.9, 24.62) -> (-11.9, 24.62)
  line L142 (-11.9, 24.62) -> (-11.9, 25.62)
  line L143 (-11.9, 25.62) -> (-10.9, 25.62)
  line L144 (-10.9, 22.99) -> (-10.9, 21.99)
  line L145 (-10.9, 21.99) -> (-11.9, 21.99)
  line L146 (-11.9, 21.99) -> (-11.9, 22.99)
  line L147 (-11.9, 22.99) -> (-10.9, 22.99)
  line L148 (-10.9, 20.36) -> (-10.9, 19.36)
  line L149 (-10.9, 19.36) -> (-11.9, 19.36)
  line L150 (-11.9, 19.36) -> (-11.9, 20.36)
  line L151 (-11.9, 20.36) -> (-10.9, 20.36)
  line L152 (-10.9, 17.73) -> (-10.9, 16.73)
  line L153 (-10.9, 16.73) -> (-11.9, 16.73)
  line L154 (-11.9, 16.73) -> (-11.9, 17.73)
  line L155 (-11.9, 17.73) -> (-10.9, 17.73)
  line L156 (-10.9, 15.1) -> (-10.9, 14.1)
  line L157 (-10.9, 14.1) -> (-11.9, 14.1)
  line L158 (-11.9, 14.1) -> (-11.9, 15.1)
  line L159 (-11.9, 15.1) -> (-10.9, 15.1)
  line L160 (-10.9, 12.47) -> (-10.9, 11.47)
  line L161 (-10.9, 11.47) -> (-11.9, 11.47)
  line L162 (-11.9, 11.47) -> (-11.9, 12.47)
  line L163 (-11.9, 12.47) -> (-10.9, 12.47)
  line L164 (-10.9, 9.84) -> (-10.9, 8.84)
  line L165 (-10.9, 8.84) -> (-11.9, 8.84)
  line L166 (-11.9, 8.84) -> (-11.9, 9.84)
  line L167 (-11.9, 9.84) -> (-10.9, 9.84)
  line L168 (-10.9, 7.21) -> (-10.9, 6.21)
  line L169 (-10.9, 6.21) -> (-11.9, 6.21)
  line L170 (-11.9, 6.21) -> (-11.9, 7.21)
  line L171 (-11.9, 7.21) -> (-10.9, 7.21)
  line L172 (-10.9, 4.58) -> (-10.9, 3.58)
  line L173 (-10.9, 3.58) -> (-11.9, 3.58)
  line L174 (-11.9, 3.58) -> (-11.9, 4.58)
  line L175 (-11.9, 4.58) -> (-10.9, 4.58)
  line L176 (-10.9, 1.95) -> (-10.9, 0.95)
  line L177 (-10.9, 0.95) -> (-11.9, 0.95)
  line L178 (-11.9, 0.95) -> (-11.9, 1.95)
  line L179 (-11.9, 1.95) -> (-10.9, 1.95)
  line L180 (-10.9, -0.68) -> (-10.9, -1.68)
  line L181 (-10.9, -1.68) -> (-11.9, -1.68)
  line L182 (-11.9, -1.68) -> (-11.9, -0.68)
  line L183 (-11.9, -0.68) -> (-10.9, -0.68)
  line L184 (-10.9, -3.31) -> (-10.9, -4.31)
  line L185 (-10.9, -4.31) -> (-11.9, -4.31)
  line L186 (-11.9, -4.31) -> (-11.9, -3.31)
  line L187 (-11.9, -3.31) -> (-10.9, -3.31)
  line L188 (-10.9, -5.94) -> (-10.9, -6.94)
  line L189 (-10.9, -6.94) -> (-11.9, -6.94)
  line L190 (-11.9, -6.94) -> (-11.9, -5.94)
  line L191 (-11.9, -5.94) -> (-10.9, -5.94)
  line L192 (-10.9, -8.57) -> (-10.9, -9.57)
  line L193 (-10.9, -9.57) -> (-11.9, -9.57)
  line L194 (-11.9, -9.57) -> (-11.9, -8.57)
  line L195 (-11.9, -8.57) -> (-10.9, -8.57)
  line L196 (-10.9, -11.2) -> (-10.9, -12.2)
  line L197 (-10.9, -12.2) -> (-11.9, -12.2)
  line L198 (-11.9, -12.2) -> (-11.9, -11.2)
  line L199 (-11.9, -11.2) -> (-10.9, -11.2)
  line L200 (-10.9, -13.83) -> (-10.9, -14.83)
  line L201 (-10.9, -14.83) -> (-11.9, -14.83)
  line L202 (-11.9, -14.83) -> (-11.9, -13.83)
  line L203 (-11.9, -13.83) -> (-10.9, -13.83)
  line L204 (-10.9, -16.46) -> (-10.9, -17.46)
  line L205 (-10.9, -17.46) -> (-11.9, -17.46)
  line L206 (-11.9, -17.46) -> (-11.9, -16.46)
  line L207 (-11.9, -16.46) -> (-10.9, -16.46)
  line L208 (-10.9, -19.09) -> (-10.9, -20.09)
  line L209 (-10.9, -20.09) -> (-11.9, -20.09)
  line L210 (-11.9, -20.09) -> (-11.9, -19.09)
  line L211 (-11.9, -19.09) -> (-10.9, -19.09)
  line L212 (-10.9, -21.72) -> (-10.9, -22.72)
  line L213 (-10.9, -22.72) -> (-11.9, -22.72)
  line L214 (-11.9, -22.72) -> (-11.9, -21.72)
  line L215 (-11.9, -21.72) -> (-10.9, -21.72)
  line L216 (-10.9, -24.35) -> (-10.9, -25.35)
  line L217 (-10.9, -25.35) -> (-11.9, -25.35)
  line L218 (-11.9, -25.35) -> (-11.9, -24.35)
  line L219 (-11.9, -24.35) -> (-10.9, -24.35)
  line L220 (-10.9, -26.98) -> (-10.9, -27.98)
  line L221 (-10.9, -27.98) -> (-11.9, -27.98)
  line L222 (-11.9, -27.98) -> (-11.9, -26.98)
  line L223 (-11.9, -26.98) -> (-10.9, -26.98)
  line L224 (-10.9, -29.61) -> (-10.9, -30.61)
  line L225 (-10.9, -30.61) -> (-11.9, -30.61)
  line L226 (-11.9, -30.61) -> (-11.9, -29.61)
  line L227 (-11.9, -29.61) -> (-10.9, -29.61)
  line L228 (-10.9, -32.24) -> (-10.9, -33.24)
  line L229 (-10.9, -33.24) -> (-11.9, -33.24)
  line L230 (-11.9, -33.24) -> (-11.9, -32.24)
  line L231 (-11.9, -32.24) -> (-10.9, -32.24)
  line L232 (-10.9, -34.87) -> (-10.9, -35.87)
  line L233 (-10.9, -35.87) -> (-11.9, -35.87)
  line L234 (-11.9, -35.87) -> (-11.9, -34.87)
  line L235 (-11.9, -34.87) -> (-10.9, -34.87)
  line L236 (-10.9, -37.5) -> (-10.9, -38.5)
  line L237 (-10.9, -38.5) -> (-11.9, -38.5)
  line L238 (-11.9, -38.5) -> (-11.9, -37.5)
  line L239 (-11.9, -37.5) -> (-10.9, -37.5)
  line L240 (-8.1, 38.77) -> (-8.1, 37.77)
  line L241 (-8.1, 37.77) -> (-9.1, 37.77)
  line L242 (-9.1, 37.77) -> (-9.1, 38.77)
  line L243 (-9.1, 38.77) -> (-8.1, 38.77)
  line L244 (-8.1, 36.14) -> (-8.1, 35.14)
  line L245 (-8.1, 35.14) -> (-9.1, 35.14)
  line L246 (-9.1, 35.14) -> (-9.1, 36.14)
  line L247 (-9.1, 36.14) -> (-8.1, 36.14)
  line L248 (-8.1, 33.51) -> (-8.1, 32.51)
  line L249 (-8.1, 32.51) -> (-9.1, 32.51)
  line L250 (-9.1, 32.51) -> (-9.1, 33.51)
  line L251 (-9.1, 33.51) -> (-8.1, 33.51)
  line L252 (-8.1, 30.88) -> (-8.1, 29.88)
  line L253 (-8.1, 29.88) -> (-9.1, 29.88)
  line L254 (-9.1, 29.88) -> (-9.1, 30.88)
  line L255 (-9.1, 30.88) -> (-8.1, 30.88)
  line L256 (-8.1, 28.25) -> (-8.1, 27.25)
  line L257 (-8.1, 27.25) -> (-9.1, 27.25)
  line L258 (-9.1, 27.25) -> (-9.1, 28.25)
  line L259 (-9.1, 28.25) -> (-8.1, 28.25)
  line L260 (-8.1, 25.62) -> (-8.1, 24.62)
  line L261 (-8.1, 24.62) -> (-9.1, 24.62)
  line L262 (-9.1, 24.62) -> (-9.1, 25.62)
  line L263 (-9.1, 25.62) -> (-8.1, 25.62)
  line L264 (-8.1, 22.99) -> (-8.1, 21.99)
  line L265 (-8.1, 21.99) -> (-9.1, 21.99)
  line L266 (-9.1, 21.99) -> (-9.1, 22.99)
  line L267 (-9.1, 22.99) -> (-8.1, 22.99)
  line L268 (-8.1, 20.36) -> (-8.1, 19.36)
  line L269 (-8.1, 19.36) -> (-9.1, 19.36)
  line L270 (-9.1, 19.36) -> (-9.1, 20.36)
  line L271 (-9.1, 20.36) -> (-8.1, 20.36)
  line L272 (-8.1, 17.73) -> (-8.1, 16.73)
  line L273 (-8.1, 16.73) -> (-9.1, 16.73)
  line L274 (-9.1, 16.73) -> (-9.1, 17.73)
  line L275 (-9.1, 17.73) -> (-8.1, 17.73)
  line L276 (-8.1, 15.1) -> (-8.1, 14.1)
  line L277 (-8.1, 14.1) -> (-9.1, 14.1)
  line L278 (-9.1, 14.1) -> (-9.1, 15.1)
  line L279 (-9.1, 15.1) -> (-8.1, 15.1)
  line L280 (-8.1, 12.47) -> (-8.1, 11.47)
  line L281 (-8.1, 11.47) -> (-9.1, 11.47)
  line L282 (-9.1, 11.47) -> (-9.1, 12.47)
  line L283 (-9.1, 12.47) -> (-8.1, 12.47)
  line L284 (-8.1, 9.84) -> (-8.1, 8.84)
  line L285 (-8.1, 8.84) -> (-9.1, 8.84)
  line L286 (-9.1, 8.84) -> (-9.1, 9.84)
  line L287 (-9.1, 9.84) -> (-8.1, 9.84)
  line L288 (-8.1, 7.21) -> (-8.1, 6.21)
  line L289 (-8.1, 6.21) -> (-9.1, 6.21)
  line L290 (-9.1, 6.21) -> (-9.1, 7.21)
  line L291 (-9.1, 7.21) -> (-8.1, 7.21)
  line L292 (-8.1, 4.58) -> (-8.1, 3.58)
  line L293 (-8.1, 3.58) -> (-9.1, 3.58)
  line L294 (-9.1, 3.58) -> (-9.1, 4.58)
  line L295 (-9.1, 4.58) -> (-8.1, 4.58)
  line L296 (-8.1, 1.95) -> (-8.1, 0.95)
  line L297 (-8.1, 0.95) -> (-9.1, 0.95)
  line L298 (-9.1, 0.95) -> (-9.1, 1.95)
  line L299 (-9.1, 1.95) -> (-8.1, 1.95)
  line L300 (-8.1, -0.68) -> (-8.1, -1.68)
  line L301 (-8.1, -1.68) -> (-9.1, -1.68)
  line L302 (-9.1, -1.68) -> (-9.1, -0.68)
  line L303 (-9.1, -0.68) -> (-8.1, -0.68)
  line L304 (-8.1, -3.31) -> (-8.1, -4.31)
  line L305 (-8.1, -4.31) -> (-9.1, -4.31)
  line L306 (-9.1, -4.31) -> (-9.1, -3.31)
  line L307 (-9.1, -3.31) -> (-8.1, -3.31)
  line L308 (-8.1, -5.94) -> (-8.1, -6.94)
  line L309 (-8.1, -6.94) -> (-9.1, -6.94)
  line L310 (-9.1, -6.94) -> (-9.1, -5.94)
  line L311 (-9.1, -5.94) -> (-8.1, -5.94)
  line L312 (-8.1, -8.57) -> (-8.1, -9.57)
  line L313 (-8.1, -9.57) -> (-9.1, -9.57)
  line L314 (-9.1, -9.57) -> (-9.1, -8.57)
  line L315 (-9.1, -8.57) -> (-8.1, -8.57)
  line L316 (-8.1, -11.2) -> (-8.1, -12.2)
  line L317 (-8.1, -12.2) -> (-9.1, -12.2)
  line L318 (-9.1, -12.2) -> (-9.1, -11.2)
  line L319 (-9.1, -11.2) -> (-8.1, -11.2)
  line L320 (-8.1, -13.83) -> (-8.1, -14.83)
  line L321 (-8.1, -14.83) -> (-9.1, -14.83)
  line L322 (-9.1, -14.83) -> (-9.1, -13.83)
  line L323 (-9.1, -13.83) -> (-8.1, -13.83)
  line L324 (-8.1, -16.46) -> (-8.1, -17.46)
  line L325 (-8.1, -17.46) -> (-9.1, -17.46)
  line L326 (-9.1, -17.46) -> (-9.1, -16.46)
  line L327 (-9.1, -16.46) -> (-8.1, -16.46)
  line L328 (-8.1, -19.09) -> (-8.1, -20.09)
  line L329 (-8.1, -20.09) -> (-9.1, -20.09)
  line L330 (-9.1, -20.09) -> (-9.1, -19.09)
  line L331 (-9.1, -19.09) -> (-8.1, -19.09)
  line L332 (-8.1, -21.72) -> (-8.1, -22.72)
  line L333 (-8.1, -22.72) -> (-9.1, -22.72)
  line L334 (-9.1, -22.72) -> (-9.1, -21.72)
  line L335 (-9.1, -21.72) -> (-8.1, -21.72)
  line L336 (-8.1, -24.35) -> (-8.1, -25.35)
  line L337 (-8.1, -25.35) -> (-9.1, -25.35)
  line L338 (-9.1, -25.35) -> (-9.1, -24.35)
  line L339 (-9.1, -24.35) -> (-8.1, -24.35)
  line L340 (-8.1, -26.98) -> (-8.1, -27.98)
  line L341 (-8.1, -27.98) -> (-9.1, -27.98)
  line L342 (-9.1, -27.98) -> (-9.1, -26.98)
  line L343 (-9.1, -26.98) -> (-8.1, -26.98)
  line L344 (-8.1, -29.61) -> (-8.1, -30.61)
  line L345 (-8.1, -30.61) -> (-9.1, -30.61)
  line L346 (-9.1, -30.61) -> (-9.1, -29.61)
  line L347 (-9.1, -29.61) -> (-8.1, -29.61)
  line L348 (-8.1, -32.24) -> (-8.1, -33.24)
  line L349 (-8.1, -33.24) -> (-9.1, -33.24)
  line L350 (-9.1, -33.24) -> (-9.1, -32.24)
  line L351 (-9.1, -32.24) -> (-8.1, -32.24)
  line L352 (-8.1, -34.87) -> (-8.1, -35.87)
  line L353 (-8.1, -35.87) -> (-9.1, -35.87)
  line L354 (-9.1, -35.87) -> (-9.1, -34.87)
  line L355 (-9.1, -34.87) -> (-8.1, -34.87)
  line L356 (-8.1, -37.5) -> (-8.1, -38.5)
  line L357 (-8.1, -38.5) -> (-9.1, -38.5)
  line L358 (-9.1, -38.5) -> (-9.1, -37.5)
  line L359 (-9.1, -37.5) -> (-8.1, -37.5)
  line L360 (-5.3, 38.77) -> (-5.3, 37.77)
  line L361 (-5.3, 37.77) -> (-6.3, 37.77)
  line L362 (-6.3, 37.77) -> (-6.3, 38.77)
  line L363 (-6.3, 38.77) -> (-5.3, 38.77)
  line L364 (-5.3, 36.14) -> (-5.3, 35.14)
  line L365 (-5.3, 35.14) -> (-6.3, 35.14)
  line L366 (-6.3, 35.14) -> (-6.3, 36.14)
  line L367 (-6.3, 36.14) -> (-5.3, 36.14)
  line L368 (-5.3, 33.51) -> (-5.3, 32.51)
  line L369 (-5.3, 32.51) -> (-6.3, 32.51)
  line L370 (-6.3, 32.51) -> (-6.3, 33.51)
  line L371 (-6.3, 33.51) -> (-5.3, 33.51)
  line L372 (-5.3, 30.88) -> (-5.3, 29.88)
  line L373 (-5.3, 29.88) -> (-6.3, 29.88)
  line L374 (-6.3, 29.88) -> (-6.3, 30.88)
  line L375 (-6.3, 30.88) -> (-5.3, 30.88)
  line L376 (-5.3, 28.25) -> (-5.3, 27.25)
  line L377 (-5.3, 27.25) -> (-6.3, 27.25)
  line L378 (-6.3, 27.25) -> (-6.3, 28.25)
  line L379 (-6.3, 28.25) -> (-5.3, 28.25)
  line L380 (-5.3, 25.62) -> (-5.3, 24.62)
  line L381 (-5.3, 24.62) -> (-6.3, 24.62)
  line L382 (-6.3, 24.62) -> (-6.3, 25.62)
  line L383 (-6.3, 25.62) -> (-5.3, 25.62)
  line L384 (-5.3, 22.99) -> (-5.3, 21.99)
  line L385 (-5.3, 21.99) -> (-6.3, 21.99)
  line L386 (-6.3, 21.99) -> (-6.3, 22.99)
  line L387 (-6.3, 22.99) -> (-5.3, 22.99)
  line L388 (-5.3, 20.36) -> (-5.3, 19.36)
  line L389 (-5.3, 19.36) -> (-6.3, 19.36)
  line L390 (-6.3, 19.36) -> (-6.3, 20.36)
  line L391 (-6.3, 20.36) -> (-5.3, 20.36)
  line L392 (-5.3, 17.73) -> (-5.3, 16.73)
  line L393 (-5.3, 16.73) -> (-6.3, 16.73)
  line L394 (-6.3, 16.73) -> (-6.3, 17.73)
  line L395 (-6.3, 17.73) -> (-5.3, 17.73)
  line L396 (-5.3, 15.1) -> (-5.3, 14.1)
  line L397 (-5.3, 14.1) -> (-6.3, 14.1)
  line L398 (-6.3, 14.1) -> (-6.3, 15.1)
  line L399 (-6.3, 15.1) -> (-5.3, 15.1)
  line L400 (-5.3, 12.47) -> (-5.3, 11.47)
  line L401 (-5.3, 11.47) -> (-6.3, 11.47)
  line L402 (-6.3, 11.47) -> (-6.3, 12.47)
  line L403 (-6.3, 12.47) -> (-5.3, 12.47)
  line L404 (-5.3, 9.84) -> (-5.3, 8.84)
  line L405 (-5.3, 8.84) -> (-6.3, 8.84)
  line L406 (-6.3, 8.84) -> (-6.3, 9.84)
  line L407 (-6.3, 9.84) -> (-5.3, 9.84)
  line L408 (-5.3, 7.21) -> (-5.3, 6.21)
  line L409 (-5.3, 6.21) -> (-6.3, 6.21)
  line L410 (-6.3, 6.21) -> (-6.3, 7.21)
  line L411 (-6.3, 7.21) -> (-5.3, 7.21)
  line L412 (-5.3, 4.58) -> (-5.3, 3.58)
  line L413 (-5.3, 3.58) -> (-6.3, 3.58)
  line L414 (-6.3, 3.58) -> (-6.3, 4.58)
  line L415 (-6.3, 4.58) -> (-5.3, 4.58)
  line L416 (-5.3, 1.95) -> (-5.3, 0.95)
  line L417 (-5.3, 0.95) -> (-6.3, 0.95)
  line L418 (-6.3, 0.95) -> (-6.3, 1.95)
  line L419 (-6.3, 1.95) -> (-5.3, 1.95)
  line L420 (-5.3, -0.68) -> (-5.3, -1.68)
  line L421 (-5.3, -1.68) -> (-6.3, -1.68)
  line L422 (-6.3, -1.68) -> (-6.3, -0.68)
  line L423 (-6.3, -0.68) -> (-5.3, -0.68)
  line L424 (-5.3, -3.31) -> (-5.3, -4.31)
  line L425 (-5.3, -4.31) -> (-6.3, -4.31)
  line L426 (-6.3, -4.31) -> (-6.3, -3.31)
  line L427 (-6.3, -3.31) -> (-5.3, -3.31)
  line L428 (-5.3, -5.94) -> (-5.3, -6.94)
  line L429 (-5.3, -6.94) -> (-6.3, -6.94)
  line L430 (-6.3, -6.94) -> (-6.3, -5.94)
  line L431 (-6.3, -5.94) -> (-5.3, -5.94)
  line L432 (-5.3, -8.57) -> (-5.3, -9.57)
  line L433 (-5.3, -9.57) -> (-6.3, -9.57)
  line L434 (-6.3, -9.57) -> (-6.3, -8.57)
  line L435 (-6.3, -8.57) -> (-5.3, -8.57)
  line L436 (-5.3, -11.2) -> (-5.3, -12.2)
  line L437 (-5.3, -12.2) -> (-6.3, -12.2)
  line L438 (-6.3, -12.2) -> (-6.3, -11.2)
  line L439 (-6.3, -11.2) -> (-5.3, -11.2)
  line L440 (-5.3, -13.83) -> (-5.3, -14.83)
  line L441 (-5.3, -14.83) -> (-6.3, -14.83)
  line L442 (-6.3, -14.83) -> (-6.3, -13.83)
  line L443 (-6.3, -13.83) -> (-5.3, -13.83)
  line L444 (-5.3, -16.46) -> (-5.3, -17.46)
  line L445 (-5.3, -17.46) -> (-6.3, -17.46)
  line L446 (-6.3, -17.46) -> (-6.3, -16.46)
  line L447 (-6.3, -16.46) -> (-5.3, -16.46)
  line L448 (-5.3, -19.09) -> (-5.3, -20.09)
  line L449 (-5.3, -20.09) -> (-6.3, -20.09)
  line L450 (-6.3, -20.09) -> (-6.3, -19.09)
  line L451 (-6.3, -19.09) -> (-5.3, -19.09)
  line L452 (-5.3, -21.72) -> (-5.3, -22.72)
  line L453 (-5.3, -22.72) -> (-6.3, -22.72)
  line L454 (-6.3, -22.72) -> (-6.3, -21.72)
  line L455 (-6.3, -21.72) -> (-5.3, -21.72)
  line L456 (-5.3, -24.35) -> (-5.3, -25.35)
  line L457 (-5.3, -25.35) -> (-6.3, -25.35)
  line L458 (-6.3, -25.35) -> (-6.3, -24.35)
  line L459 (-6.3, -24.35) -> (-5.3, -24.35)
  line L460 (-5.3, -26.98) -> (-5.3, -27.98)
  line L461 (-5.3, -27.98) -> (-6.3, -27.98)
  line L462 (-6.3, -27.98) -> (-6.3, -26.98)
  line L463 (-6.3, -26.98) -> (-5.3, -26.98)
  line L464 (-5.3, -29.61) -> (-5.3, -30.61)
  line L465 (-5.3, -30.61) -> (-6.3, -30.61)
  line L466 (-6.3, -30.61) -> (-6.3, -29.61)
  line L467 (-6.3, -29.61) -> (-5.3, -29.61)
  line L468 (-5.3, -32.24) -> (-5.3, -33.24)
  line L469 (-5.3, -33.24) -> (-6.3, -33.24)
  line L470 (-6.3, -33.24) -> (-6.3, -32.24)
  line L471 (-6.3, -32.24) -> (-5.3, -32.24)
  line L472 (-5.3, -34.87) -> (-5.3, -35.87)
  line L473 (-5.3, -35.87) -> (-6.3, -35.87)
  line L474 (-6.3, -35.87) -> (-6.3, -34.87)
  line L475 (-6.3, -34.87) -> (-5.3, -34.87)
  line L476 (-5.3, -37.5) -> (-5.3, -38.5)
  line L477 (-5.3, -38.5) -> (-6.3, -38.5)
  line L478 (-6.3, -38.5) -> (-6.3, -37.5)
  line L479 (-6.3, -37.5) -> (-5.3, -37.5)
  line L480 (-2.5, 38.77) -> (-2.5, 37.77)
  line L481 (-2.5, 37.77) -> (-3.5, 37.77)
  line L482 (-3.5, 37.77) -> (-3.5, 38.77)
  line L483 (-3.5, 38.77) -> (-2.5, 38.77)
  line L484 (-2.5, 36.14) -> (-2.5, 35.14)
  line L485 (-2.5, 35.14) -> (-3.5, 35.14)
  line L486 (-3.5, 35.14) -> (-3.5, 36.14)
  line L487 (-3.5, 36.14) -> (-2.5, 36.14)
  line L488 (-2.5, 33.51) -> (-2.5, 32.51)
  line L489 (-2.5, 32.51) -> (-3.5, 32.51)
  line L490 (-3.5, 32.51) -> (-3.5, 33.51)
  line L491 (-3.5, 33.51) -> (-2.5, 33.51)
  line L492 (-2.5, 30.88) -> (-2.5, 29.88)
  line L493 (-2.5, 29.88) -> (-3.5, 29.88)
  line L494 (-3.5, 29.88) -> (-3.5, 30.88)
  line L495 (-3.5, 30.88) -> (-2.5, 30.88)
  line L496 (-2.5, 28.25) -> (-2.5, 27.25)
  line L497 (-2.5, 27.25) -> (-3.5, 27.25)
  line L498 (-3.5, 27.25) -> (-3.5, 28.25)
  line L499 (-3.5, 28.25) -> (-2.5, 28.25)
  line L500 (-2.5, 25.62) -> (-2.5, 24.62)
  line L501 (-2.5, 24.62) -> (-3.5, 24.62)
  line L502 (-3.5, 24.62) -> (-3.5, 25.62)
  line L503 (-3.5, 25.62) -> (-2.5, 25.62)
  line L504 (-2.5, 22.99) -> (-2.5, 21.99)